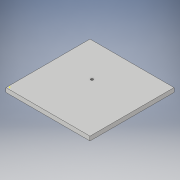
# Autodesk Inventor part: base
Saved by Autodesk Inventor 2019 (Build 230136000, 136)
## iProperties
Created: 2020-02-20
Part Number: base
Material: Generic
Document SubType Name: Modeling
Designer: ADMIN
Density: 1 g/cm^3
Appearance: Default
Author: ADMIN
Autodesk Inventor part; units mm, degrees
ref_plane "YZ Plane" through (0, 0, 0) normal (1, 0, 0) x (0, 1, 0)
ref_plane "XZ Plane" through (0, 0, 0) normal (0, 1, 0) x (-1, 0, 0)
ref_plane "XY Plane" through (0, 0, 0) normal (0, 0, 1) x (1, 0, 0)
sketch "Sketch1" plane through (0, 0, 0) normal (0, 1, 0) x (-1, 0, 0)
  line L0 (11.7573, 15.6474) -> (-588.2427, 15.6474)
  line L1 (-588.2427, 15.6474) -> (-588.2427, -584.3526)
  line L2 (-588.2427, -584.3526) -> (11.7573, -584.3526)
  line L3 (11.7573, -584.3526) -> (11.7573, 15.6474)
  point P0 (0, 0)
  dimension "d0" = 600
  dimension "d1" = 600
  dimension "d2" = 600
  dimension "d3" = 600
  constraints: 8 end point, 2 perpendicular, 1 horizontal
  measures "d0" distance of L0.start L0.end
  measures "d1" distance of L0.end L1.end
  measures "d2" distance of L1.end L2.end
  measures "d3" distance of L2.end L0.start
extrude "Extrusion1" add sketch "Sketch1" along normal blind 30
sketch "Sketch2" plane through (0, 30, 0) normal (0, 1, 0) x (1, 0, 0)
  point P0 (0, 0)
sketch "Sketch3" plane through (0, 30, 0) normal (0, 1, 0) x (1, 0, 0)
  point P0 (0, 0)
  point P1 (244.8826, 341.7694)
hole "Hole1" at (244.8826, 30, -341.7694) direction (0, -1, 0) diameter 17.894 depth 53.975 tip angle 118 thread size "13/16-10 UNC" class "2B" standard "ANSI Unified Screw Threads"
body "Solid1"
